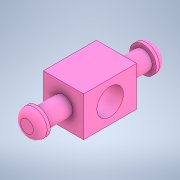
# Autodesk Inventor part: Insert
Saved by Autodesk Inventor 2022.4 (Build 264492000, 492)
## iProperties
Created: 2024-04-25
Part Number: Insert
Material: Generic
Document SubType Name: Modeling
Designer: t60147996
Density: 1 g/cm^3
Appearance: Pink
Author: t60147996
Autodesk Inventor part; units mm, degrees
ref_plane "YZ Plane" through (0, 0, 0) normal (1, 0, 0) x (0, 1, 0)
ref_plane "XZ Plane" through (0, 0, 0) normal (0, 1, 0) x (-1, 0, 0)
ref_plane "XY Plane" through (0, 0, 0) normal (0, 0, 1) x (1, 0, 0)
sketch "Sketch1" plane through (0, 0, 0) normal (0, 0, 1) x (1, 0, 0)
  circle A0 centre (0, 0) radius 4.445
  dimension "d0" = 8.89
  constraints: 1 centre point, 1 coincident
  measures "d0" diameter of A0
extrude "Extrusion1" add sketch "Sketch1" along normal mid plane 50.8
sketch "Sketch2" plane through (0, 0, 25.4) normal (0, 0, 1) x (1, 0, 0)
  circle A0 centre (0, 0) radius 6.35
  dimension "d3" = 12.7
  constraints: 1 centre point, 1 coincident
  measures "d3" diameter of A0
extrude "Extrusion2" add sketch "Sketch2" along normal blind 4.826
fillet "Fillet1" radius 3.302 1 edges at (-6.35, 0, 30.226)
mirror "Mirror1" about plane through (0, 0, 0) normal (0, 0, 1) of "Extrusion2", "Fillet1"
sketch "Sketch3" plane through (0, 0, 0) normal (1, 0, 0) x (0, 1, 0)
  line L0 (-9.525, -12.7) -> (9.525, -12.7)
  line L1 (9.525, -12.7) -> (9.525, 12.7)
  line L2 (9.525, 12.7) -> (-9.525, 12.7)
  line L3 (-9.525, 12.7) -> (-9.525, -12.7)
  line L4 (-9.525, -12.7) -> (9.525, 12.7) construction
  line L5 (9.525, -12.7) -> (-9.525, 12.7) construction
  point P0 (0, 0)
  dimension "d7" = 19.05
  dimension "d8" = 25.4
  constraints: 12 end point, 2 midpoint, 2 parallel, 1 horizontal, 1 perpendicular
  measures "d7" distance of L2.end L1.end
  measures "d8" distance of L1.end L0.end
extrude "Extrusion3" add sketch "Sketch3" along normal mid plane 19.304
sketch "Sketch4" plane through (9.652, 0, 0) normal (1, 0, 0) x (0, 0, -1)
  point P0 (0, 0)
  point P1 (0, 0)
  constraints: 1 coincident
hole "Hole1" at (9.652, 0, 0) direction (-1, 0, 0) diameter 12.7 end through all
body "Solid1"
